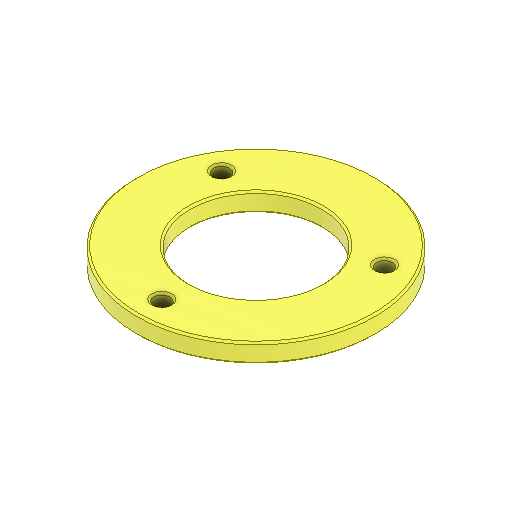
# Autodesk Inventor part: B_probe_bearing_without_holes
Saved by Autodesk Inventor 2026.2 (Build 302298000, 298)
## iProperties
Created: 2026-06-04
Part Number: B_probe_bearing_without_holes
Material: PAEK 樹脂
Document SubType Name: Modeling
Designer: zetsu
Density: 1.32 g/cm^3
Appearance: 滑らか - 黄
Author: zetsu
Autodesk Inventor part; units mm, degrees
ref_plane "YZ Plane" through (0, 0, 0) normal (1, 0, 0) x (0, 1, 0)
ref_plane "XZ Plane" through (0, 0, 0) normal (0, 1, 0) x (-1, 0, 0)
ref_plane "XY Plane" through (0, 0, 0) normal (0, 0, 1) x (1, 0, 0)
sketch "スケッチ1" plane through (0, 0, 0) normal (0, 1, 0) x (-1, 0, 0)
  circle A0 centre (0, 0) radius 31.75
  dimension "d0" = 63.5
  constraints: 1 centre point, 1 coincident
  measures "d0" diameter of A0
extrude "押し出し1" add sketch "スケッチ1" along normal blind 5
sketch "スケッチ4" plane through (0, 5, 0) normal (0, 1, 0) x (1, 0, 0)
  circle A0 centre (0, 0) radius 17.5
  dimension "d9" = 35
  constraints: 1 centre point, 1 coincident
  measures "d9" diameter of A0
extrude "押し出し4" cut sketch "スケッチ4" against normal through all
sketch "スケッチ6" plane through (0, 5, 0) normal (0, 1, 0) x (1, 0, 0)
  circle A0 centre (0, 0) radius 25 construction
  circle A1 centre (21.6506, 12.5) radius 2.15
  line L0 (0, 0) -> (21.6506, 12.5) construction
  line L1 (0, 0) -> (35.9214, 0) construction
  circle A2 centre (-21.6506, 12.5) radius 2.15
  circle A3 centre (0, -25) radius 2.15
  dimension "d19" = 50
  dimension "d20" = 4.3
  dimension "d21" = 30
  dimension "d24" = 360
  constraints: 4 end point, 3 centre point, 1 coincident, 1 horizontal, 10 other
  measures "d20" diameter of A1
  measures "d21" angle of L1 L0
extrude "押し出し6" cut sketch "スケッチ6" against normal through all
chamfer "面取り1" distance 0.5 angle 45 10 edges at (31.75, 5, 0) (31.75, 0, 0) (-23.8006, 5, -12.5) (-2.15, 5, 25) (19.5006, 5, -12.5) (-17.5, 5, 0) (-17.5, 0, 0) (-23.8006, 0, -12.5) (-2.15, 0, 25) (19.5006, 0, -12.5)
